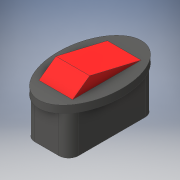
# Autodesk Inventor part: SwitchRocker
Saved by Autodesk Inventor 2016 (Build 200138000, 138)
## iProperties
Created: 2015-10-16
Part Number: SwitchRocker
Material: Generic
Document SubType Name: Modeling
Designer: lachesis
Density: 1 g/cm^3
Appearance: Default
Author: lachesis
Autodesk Inventor part; units mm, degrees
ref_plane "YZ Plane" through (0, 0, 0) normal (1, 0, 0) x (0, 1, 0)
ref_plane "XZ Plane" through (0, 0, 0) normal (0, 1, 0) x (-1, 0, 0)
ref_plane "XY Plane" through (0, 0, 0) normal (0, 0, 1) x (1, 0, 0)
sketch "Sketch1" plane through (0, 0, 0) normal (0, 1, 0) x (-1, 0, 0)
  line L0 (8.9, 17.6) -> (-8.9, 17.6)
  line L1 (-8.9, 17.6) -> (-8.9, -17.6)
  line L2 (-8.9, -17.6) -> (8.9, -17.6)
  line L3 (8.9, -17.6) -> (8.9, 17.6)
  point P0 (0, 0)
  point P1 (8.9, 0)
  point P2 (0, -17.6)
  dimension "d0" = 35.2
  dimension "d1" = 17.8
  constraints: 8 end point, 2 midpoint, 2 parallel, 1 horizontal, 1 horizontal alignment, 1 perpendicular, 1 vertical alignment
  measures "d0" distance of L2.end L0.start
  measures "d1" distance of L1.end L2.end
extrude "Extrusion1" add sketch "Sketch1" along normal blind 16
sketch "Sketch2" plane through (0, 16, 0) normal (0, 1, 0) x (1, 0, 0)
  ellipse E0 centre (0, 0) end of major axis (0, 21) minor radius 13
  dimension "d4" = 21
  dimension "d5" = 13
  constraints: 1 coincident, 2 other
extrude "Extrusion2" add sketch "Sketch2" along normal blind 3
fillet "Fillet1" radius 4 4 edges at (8.9, 8, 17.6) (8.9, 8, -17.6) (-8.9, 8, 17.6) (-8.9, 8, -17.6)
ref_plane "Work Plane1" through (6.9, 0, 13.6) normal (1, 0, 0) x (0, 0, -1)
sketch "Sketch3" plane through (6.9, 0, 13.6) normal (1, 0, 0) x (0, 0, -1)
  line L0 (34.6, 19) -> (-7.4, 19) projected
  line L1 (27.6, 19) -> (6.5786, 24)
  line L2 (6.5786, 24) -> (-0.4, 19)
  line L3 (-0.4, 19) -> (27.6, 19)
  point P0 (13.6, 0)
  dimension "d10" = 7
  dimension "d11" = 7
  dimension "d12" = 5
  dimension "d13" = 131
  constraints: 6 end point, 2 point on line, 1 collinear
  measures "d10" distance of L0.start L1.start
  measures "d11" distance of L0.end L2.end
  measures "d12" distance from line of L0 L1.end
  measures "d13" angle of L2 L1
extrude "Extrusion3" add sketch "Sketch3" against normal blind 13.8
body "Solid1"
